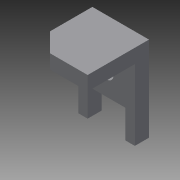
# Autodesk Inventor part: HW 2 Part 6
Saved by Autodesk Inventor 2015 (Build 190159000, 159)
## iProperties
Created: 2016-01-24
Part Number: HW 2 Part 6
Material: Generic
Document SubType Name: Modeling
Designer: Melissa
Density: 1 g/cm^3
Appearance: Default
Author: Melissa
Autodesk Inventor part; units mm, degrees
ref_plane "YZ Plane" through (0, 0, 0) normal (1, 0, 0) x (0, 1, 0)
ref_plane "XZ Plane" through (0, 0, 0) normal (0, 1, 0) x (-1, 0, 0)
ref_plane "XY Plane" through (0, 0, 0) normal (0, 0, 1) x (1, 0, 0)
sketch "Sketch1" plane through (0, 0, 0) normal (0, 0, 1) x (1, 0, 0)
  line L0 (0, 0) -> (12.7, 0)
  line L1 (12.7, 0) -> (12.7, 38.1)
  line L2 (12.7, 38.1) -> (63.5, 38.1)
  line L3 (63.5, 38.1) -> (63.5, 0)
  line L4 (63.5, 0) -> (76.2, 0)
  line L5 (76.2, 0) -> (76.2, 114.3)
  line L6 (76.2, 114.3) -> (0, 114.3)
  line L7 (0, 114.3) -> (0, 0)
  circle A0 centre (38.1, 67.818) radius 9.525
  dimension "d0" = 12.7
  dimension "d1" = 50.8
  dimension "d2" = 76.2
  dimension "d3" = 114.3
  dimension "d4" = 38.1
  dimension "d5" = 19.05
  dimension "d6" = 67.818
  dimension "d7" = 38.1
  constraints: 16 end point, 6 perpendicular, 2 point on line, 1 centre point, 1 horizontal
  measures "d0" distance of L0.start L0.end
  measures "d1" distance of L1.end L2.end
  measures "d2" distance of L5.end L6.end
  measures "d3" distance of L6.end L0.start
  measures "d4" distance of L0.end L1.end
  measures "d5" diameter of A0
  measures "d6" distance from line of L4 A0.centre
  measures "d7" distance from line of L7 A0.centre
extrude "Extrusion1" add sketch "Sketch1" against normal blind 19.05
sketch "Sketch3" plane through (0, 114.3, 0) normal (0, 1, 0) x (1, 0, 0)
  line L0 (0, 0) -> (0, -38.1)
  line L1 (0, -38.1) -> (25.4, -63.5)
  line L2 (25.4, -63.5) -> (76.2, -63.5)
  line L3 (0, 0) -> (12.7, 0) projected
  line L4 (76.2, -63.5) -> (76.2, 0)
  line L5 (76.2, 0) -> (0, 0) projected
  dimension "d10" = 90
  dimension "d11" = 90
  dimension "d12" = 50.8
  dimension "d13" = 25.4
  dimension "d14" = 63.5
  constraints: 8 end point, 1 parallel
  measures "d10" angle of L3 L0
  measures "d11" angle of L5 L4
  measures "d12" distance of L1.end L2.end
  measures "d13" horizontal distance of L0.end L1.end
  measures "d14" distance of L2.end L4.end
extrude "Extrusion2" add sketch "Sketch3" against normal blind 19.05
body "Solid1"
